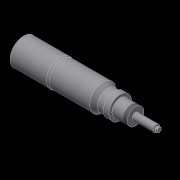
# Autodesk Inventor part: 3d_LM-Welding_Tooling -  Micrometer
Saved by Autodesk Inventor 2018.3 (Build 223284000, 284)
## iProperties
Created: 2026-01-29
Part Number: 3d_LM-Welding_Tooling -  Micrometer
Material: Genérico
Document SubType Name: Modeling
Designer: aca6
Density: 1 g/cm^3
Appearance: Valor por defecto
Author: aca6
Autodesk Inventor part; units mm, degrees
ref_plane "YZ Plane" through (0, 0, 0) normal (1, 0, 0) x (0, 1, 0)
ref_plane "XZ Plane" through (0, 0, 0) normal (0, 1, 0) x (-1, 0, 0)
ref_plane "XY Plane" through (0, 0, 0) normal (0, 0, 1) x (1, 0, 0)
sketch "Sketch6" plane through (0, 0, 0) normal (0, 0, 1) x (1, 0, 0)
  line L0 (-92.0762, 0) -> (66.22, 0)
  line L1 (-77.4867, 0) -> (-77.4867, 9.75)
  line L2 (-77.4867, 9.75) -> (-67.9253, 9.75)
  line L3 (-67.9253, 9.75) -> (-67.9253, 9.75)
  line L4 (-67.9253, 9.75) -> (-51.1938, 9.75)
  line L5 (-49.4867, 8.7929) -> (-49.4867, 0)
  line L6 (-46.409, 9.5) -> (-49.4867, 9.5)
  line L7 (-49.4867, 9.5) -> (-49.4867, 8.7929)
  line L8 (-46.409, 9.5) -> (-44.9948, 9.5) construction
  line L9 (-46.409, 9.5) -> (-20.4508, 9.5)
  line L10 (-20.4508, 9.5) -> (-16.9867, 7.5)
  line L11 (-16.9867, 7.5) -> (-11.9867, 7.5)
  line L12 (-11.9867, 7.5) -> (-11.9867, 6)
  line L13 (-11.9867, 6) -> (-3.9022, 6)
  line L14 (-3.9022, 6) -> (0.0133, 6)
  line L15 (0.0133, 6) -> (0.0133, 6)
  line L16 (0.0133, 6) -> (3.0133, 6)
  line L17 (3.0133, 6) -> (3.0133, 2.5)
  line L18 (3.0133, 2.5) -> (18.0133, 2.5)
  line L19 (18.0133, 2.5) -> (18.0133, 0)
  line L20 (-77.4867, 5.1464) -> (-79.4867, 5.1464)
  line L21 (-79.4867, 5.1464) -> (-79.4867, 0)
  line L22 (-51.1938, 9.75) -> (-49.4867, 9.5)
  line L23 (-11.9867, 7.5) -> (-11.9867, 8.2)
  line L24 (-11.9867, 8.2) -> (-7.9867, 8.2)
  line L25 (-7.9867, 8.2) -> (-7.9867, 6)
  line L26 (18.0133, 1.25) -> (19.0133, 1.25)
  line L27 (19.0133, 1.25) -> (19.0133, 0)
  point P0 (0, 0)
  dimension "d23" = 19
  dimension "d28" = 150
  dimension "d31" = 3
  dimension "d32" = 12
  dimension "d33" = 15
  dimension "d34" = 12
  dimension "d35" = 5
  dimension "d36" = 2
  dimension "d37" = 67.5
  dimension "d38" = 15
  dimension "d39" = 30
  dimension "d40" = 30
  dimension "d43" = 5
  dimension "d45" = 19.5
  dimension "d46" = 0.7
  dimension "d47" = 4
  dimension "d48" = 1
  constraints: 57 end point, 15 perpendicular, 11 point on line, 7 horizontal, 3 vertical, 1 midpoint
  measures "d23" diameter of L6 L0
  measures "d28" angle of L9 L10
  measures "d31" distance of L15.end L16.end
  measures "d32" diameter of L13 L0
  measures "d33" diameter of L11 L0
  measures "d34" diameter of L16 L0
  measures "d35" diameter of L18 L0
  measures "d36" distance of L20.start L20.end
  measures "d37" distance between parallel lines of L12 L21
  measures "d38" distance between parallel lines of L12 L17
  measures "d39" distance between parallel lines of L12 L19
  measures "d40" distance between parallel lines of L21 L5
  measures "d43" distance from line of L10.end L12
  measures "d45" diameter of L2 L0
  measures "d46" distance of L11.end L23.end
  measures "d47" distance of L23.end L24.end
  measures "d48" distance of L26.start L26.end
revolve "Revolution1" add sketch "Sketch6" angle 360 about axis through (-92.0762, 0, 0) along (1, 0, 0)
sketch "Sketch7" plane through (19.0133, 0, 0) normal (1, 0, 0) x (0, 0, -1)
  line L0 (1.7321, 0) -> (0.866, -1.5)
  line L1 (0.866, -1.5) -> (-0.866, -1.5)
  line L2 (-0.866, -1.5) -> (-1.7321, 0)
  line L3 (-1.7321, 0) -> (-0.866, 1.5)
  line L4 (-0.866, 1.5) -> (0.866, 1.5)
  line L5 (0.866, 1.5) -> (1.7321, 0)
  point P0 (0, 0)
  point P1 (0, 0)
  dimension "d49" = 3
  constraints: 12 end point, 1 coincident, 13 other
  measures "d49" distance from line of L2.end L5
extrude "Extrusion6" add sketch "Sketch7" along normal blind 1
thread "Thread1" size "M12x0.5" class "6g" standard "ISO Metric profile" length 3
body "Solid2"
